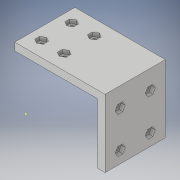
# Autodesk Inventor part: slotmountingPlate_dualcorner_m3
Saved by Autodesk Inventor 2018 (Build 220112000, 112)
## iProperties
Created: 2020-03-14
Part Number: slotmountingPlate_dualcorner_m3
Material: Generic
Document SubType Name: Modeling
Designer: natha
Density: 1 g/cm^3
Appearance: Default
Author: natha
Autodesk Inventor part; units mm, degrees
ref_plane "YZ Plane" through (0, 0, 0) normal (1, 0, 0) x (0, 1, 0)
ref_plane "XZ Plane" through (0, 0, 0) normal (0, 1, 0) x (-1, 0, 0)
ref_plane "XY Plane" through (0, 0, 0) normal (0, 0, 1) x (1, 0, 0)
sketch "Sketch1" plane through (0, 0, 0) normal (0, 1, 0) x (-1, 0, 0)
  line L0 (0, -5.4) -> (1.5, -5.4)
  line L1 (1.5, -5.4) -> (1.5, -8.1)
  line L2 (1.5, -8.1) -> (3.2, -8.1)
  line L3 (0, 0) -> (1.5, 0)
  line L4 (1.5, 0) -> (1.5, 2.7)
  line L5 (1.5, 2.7) -> (3.2, 2.7)
  line L6 (5, 0) -> (5, -5.4)
  line L7 (5, -5.4) -> (3.2, -8.1)
  line L8 (5, 0) -> (3.2, 2.7)
  line L9 (0, -20) -> (1.5, -20)
  line L10 (1.5, -20) -> (1.5, -17.3)
  line L11 (1.5, -17.3) -> (3.2, -17.3)
  line L12 (0, -25.4) -> (1.5, -25.4)
  line L13 (1.5, -25.4) -> (1.5, -28.1)
  line L14 (1.5, -28.1) -> (3.2, -28.1)
  line L15 (5, -20) -> (5, -25.4)
  line L16 (5, -25.4) -> (3.2, -28.1)
  line L17 (5, -20) -> (3.2, -17.3)
  line L18 (0, -5.4) -> (0, -20)
  line L19 (0, 0) -> (0, 7.3)
  line L20 (0, 7.3) -> (-5, 7.3)
  line L21 (0, -25.4) -> (0, -32.7)
  line L22 (0, -32.7) -> (-5, -32.7)
  line L23 (-5, -32.7) -> (-5, 7.3)
  dimension "d0" = 5.4
  dimension "d1" = 1.5
  dimension "d2" = 2.7
  dimension "d3" = 1.7
  dimension "d4" = 2.7
  dimension "d5" = 1.7
  dimension "d9" = 2.7
  dimension "d10" = 2.7
  dimension "d11" = 5.4
  dimension "d12" = 7.3
  dimension "d13" = 5
  dimension "d14" = 7.3
  dimension "d15" = 5
  dimension "d16" = 20
  constraints: 48 end point, 11 perpendicular, 4 vertical, 3 horizontal, 1 parallel
  measures "d0" distance of L3.start L0.start
  measures "d1" distance of L0.start L0.end
  measures "d2" distance of L0.end L1.end
  measures "d3" distance of L1.end L2.end
  measures "d4" distance of L3.end L4.end
  measures "d5" distance of L4.end L5.end
  measures "d9" distance of L9.end L10.end
  measures "d10" distance of L12.end L13.end
  measures "d11" distance between parallel lines of L12 L9
  measures "d12" distance of L3.start L19.end
  measures "d13" distance of L19.end L20.end
  measures "d14" distance of L12.start L21.end
  measures "d15" distance of L21.end L22.end
  measures "d16" distance between parallel lines of L3 L9
extrude "Extrusion1" add sketch "Sketch1" along normal blind 40
sketch "Sketch2" plane through (5, 0, 7.3) normal (1, 0, 0) x (0, 0, -1)
  line L0 (11.6599, 5) -> (8.3401, 5)
  line L1 (8.3401, 5) -> (6.6802, 7.875)
  line L2 (6.6802, 7.875) -> (8.3401, 10.75)
  line L3 (8.3401, 10.75) -> (11.6599, 10.75)
  line L4 (11.6599, 10.75) -> (13.3198, 7.875)
  line L5 (13.3198, 7.875) -> (11.6599, 5)
  line L6 (40, 0) -> (0, 0) projected
  line L7 (0, 0) -> (0, 40) projected
  line L8 (31.6599, 5) -> (28.3401, 5)
  line L9 (28.3401, 5) -> (26.6802, 7.875)
  line L10 (26.6802, 7.875) -> (28.3401, 10.75)
  line L11 (28.3401, 10.75) -> (31.6599, 10.75)
  line L12 (31.6599, 10.75) -> (33.3198, 7.875)
  line L13 (33.3198, 7.875) -> (31.6599, 5)
  line L14 (40, 0) -> (40, 40) projected
  line L15 (11.6599, 29.25) -> (8.3401, 29.25)
  line L16 (8.3401, 29.25) -> (6.6802, 32.125)
  line L17 (6.6802, 32.125) -> (8.3401, 35)
  line L18 (8.3401, 35) -> (11.6599, 35)
  line L19 (11.6599, 35) -> (13.3198, 32.125)
  line L20 (13.3198, 32.125) -> (11.6599, 29.25)
  line L21 (31.6599, 29.25) -> (28.3401, 29.25)
  line L22 (28.3401, 29.25) -> (26.6802, 32.125)
  line L23 (26.6802, 32.125) -> (28.3401, 35)
  line L24 (28.3401, 35) -> (31.6599, 35)
  line L25 (31.6599, 35) -> (33.3198, 32.125)
  line L26 (33.3198, 32.125) -> (31.6599, 29.25)
  line L27 (0, 40) -> (40, 40) projected
  point P0 (7.3, 0)
  point P1 (10, 7.875)
  point P2 (30, 7.875)
  point P3 (10, 32.125)
  point P4 (30, 32.125)
  dimension "d17" = 5.75
  dimension "d18" = 5
  dimension "d19" = 10
  dimension "d20" = 5.75
  dimension "d21" = 5
  dimension "d22" = 10
  dimension "d23" = 5.75
  dimension "d24" = 5.75
  dimension "d25" = 5
  dimension "d26" = 5
  dimension "d27" = 10
  dimension "d28" = 10
  constraints: 48 end point, 4 parallel, 52 other
  measures "d17" distance between parallel lines of L3 L0
  measures "d18" distance between parallel lines of L6 L0
  measures "d19" distance from line of L7 point (10, 7.875)
  measures "d20" distance between parallel lines of L11 L8
  measures "d21" distance between parallel lines of L6 L8
  measures "d22" distance from line of L14 point (30, 7.875)
  measures "d23" distance between parallel lines of L15 L18
  measures "d24" distance between parallel lines of L21 L24
  measures "d25" distance between parallel lines of L18 L27
  measures "d26" distance between parallel lines of L27 L24
  measures "d27" distance from line of L7 point (10, 32.125)
  measures "d28" distance from line of L14 point (30, 32.125)
extrude "Extrusion2" cut sketch "Sketch2" against normal blind 2.5 contours L0 L1 L2 L3 L4 L5 | L8 L9 L10 L11 L12 L13 | L15 L16 L17 L18 L19 L20 | L21 L22 L23 L24 L25 L26
sketch "Sketch3" plane through (2.5, 0, 7.3) normal (1, 0, 0) x (0, 0, -1)
  circle A0 centre (30, 7.75) radius 1.375
  circle A1 centre (10, 7.75) radius 1.375
  circle A2 centre (10, 32.25) radius 1.375
  circle A3 centre (30, 32.25) radius 1.375
  point P0 (7.3, 0)
  dimension "d31" = 2.75
  dimension "d32" = 2.75
  dimension "d33" = 2.75
  constraints: 4 centre point
  measures "d31" diameter of A0
  measures "d32" diameter of A1
  measures "d33" diameter of A2
extrude "Extrusion3" cut sketch "Sketch3" against normal blind 20
sketch "Sketch4" plane through (0, 40, 0) normal (0, 1, 0) x (1, 0, 0)
  line L0 (5, -7.3) -> (5, 32.7) projected
  line L1 (5, -7.3) -> (-55, -7.3)
  line L2 (-55, -7.3) -> (-55, 32.7)
  line L3 (-55, 32.7) -> (5, 32.7)
  line L4 (5, 32.7) -> (5, -7.3)
  point P0 (0, 0)
  dimension "d36" = 60
  constraints: 8 end point, 2 parallel, 1 horizontal, 1 perpendicular
  measures "d36" distance of L2.end L3.end
extrude "Extrusion4" add sketch "Sketch4" along normal blind 5
sketch "Sketch5" plane through (0, 40, 0) normal (0, -1, 0) x (1, 0, 0)
  line L0 (-55, -32.7) -> (-55, 7.3) projected
  line L1 (-20.2, 0) -> (-55, 0)
  line L2 (-55, 0) -> (-55, -5.4)
  line L3 (-55, -5.4) -> (-20.2, -5.4)
  line L4 (-20.2, -5.4) -> (-20.2, 0)
  line L5 (0, -5.4) -> (0, -20) projected
  line L6 (-20.2, -20) -> (-55, -20)
  line L7 (-55, -20) -> (-55, -25.4)
  line L8 (-55, -25.4) -> (-20.2, -25.4)
  line L9 (-20.2, -25.4) -> (-20.2, -20)
  point P0 (0, 0)
  dimension "d39" = 5.4
  dimension "d40" = 20.2
  dimension "d41" = 5.4
  constraints: 16 end point, 4 parallel, 2 horizontal, 2 perpendicular, 2 point on line
  measures "d39" distance of L2.end L1.end
  measures "d40" distance between parallel lines of L5 L4
  measures "d41" distance of L7.end L6.end
extrude "Extrusion5" add sketch "Sketch5" along normal blind 1.5
sketch "Sketch6" plane through (-55, 40, 7.3) normal (-1, 0, 0) x (0, 0, 1)
  point P0 (-7.3, -40)
sketch "Sketch7" plane through (-55, 40, 7.3) normal (-1, 0, 0) x (0, 0, 1)
  point P0 (-7.3, -40)
sketch "Sketch8" plane through (0, 38.5, 0) normal (0, -1, 0) x (1, 0, 0)
  line L0 (-55, -32.7) -> (-55, 7.3) projected
  line L1 (-20.2, 2.7) -> (-55, 2.7)
  line L2 (-55, 2.7) -> (-55, -8.1)
  line L3 (-55, -8.1) -> (-20.2, -8.1)
  line L4 (-20.2, -8.1) -> (-20.2, 2.7)
  line L5 (-20.2, -17.3) -> (-55, -17.3)
  line L6 (-55, -17.3) -> (-55, -28.1)
  line L7 (-55, -28.1) -> (-20.2, -28.1)
  line L8 (-20.2, -28.1) -> (-20.2, -17.3)
  line L9 (-20.2, -20) -> (-55, -20) projected
  point P0 (0, 0)
  dimension "d44" = 10.8
  dimension "d45" = 10.8
  dimension "d46" = 2.7
  constraints: 16 end point, 4 parallel, 3 point on line, 2 horizontal, 2 perpendicular
  measures "d44" distance of L2.end L1.end
  measures "d45" distance of L6.end L5.end
  measures "d46" distance between parallel lines of L9 L5
extrude "Extrusion6" add sketch "Sketch8" along normal blind 1.7 contours L0 L1 L4 L3 | L0 L9 L8 L7
sketch "Sketch9" plane through (-55, 40, 7.3) normal (-1, 0, 0) x (0, 0, 1)
  line L0 (-7.3, -4.809) -> (-12.7, -4.809)
  line L1 (-12.7, -40) -> (-12.7, 0) projected
  line L2 (-4.6, -3.2) -> (-15.4, -3.2) projected
  line L3 (-12.7, -4.809) -> (-15.4, -3.2)
  line L4 (-15.4, -3.2) -> (-4.6, -3.2)
  line L5 (-4.6, -3.2) -> (-7.3, -4.809)
  point P0 (-7.3, -40)
  dimension "d49" = 5.4
  constraints: 8 end point, 1 parallel, 1 point on line
  measures "d49" distance of L0.start L0.end
extrude "Extrusion7" add sketch "Sketch9" against normal blind 34.8
sketch "Sketch10" plane through (-55, 40, -20) normal (0, 0, 1) x (1, 0, 0)
  line L0 (34.8, -3.2) -> (0, -3.2) projected
  line L1 (0, 0) -> (0, -3.2) projected
  line L2 (34.8, -3.2) -> (0, -3.2)
  line L3 (0, -3.2) -> (0, -1.5)
  line L4 (0, -1.5) -> (34.8, -1.5)
  line L5 (34.8, -1.5) -> (34.8, -3.2)
  point P0 (55, -40)
  dimension "d52" = 1.7
  constraints: 8 end point, 2 parallel, 1 horizontal, 1 perpendicular, 1 point on line
  measures "d52" distance of L2.end L3.end
extrude "Extrusion8" add sketch "Sketch10" along normal blind 2.7
sketch "Sketch11" plane through (-55, 40, 7.3) normal (-1, 0, 0) x (0, 0, 1)
  line L0 (-24.6, -3.2) -> (-24.6, -1.5) projected
  line L1 (-35.4, -3.2) -> (-24.6, -3.2) projected
  line L2 (-24.6, -3.2) -> (-35.4, -3.2)
  line L3 (-27.3, -5) -> (-32.7, -5)
  line L4 (-32.7, -5) -> (-35.4, -3.2)
  line L5 (-24.6, -3.2) -> (-27.3, -5)
  line L6 (-27.3, 0) -> (-32.7, 0) projected
  point P0 (-7.3, -40)
  dimension "d55" = 5.4
  dimension "d56" = 5
  constraints: 8 end point, 2 horizontal
  measures "d55" distance of L3.start L3.end
  measures "d56" distance between parallel lines of L6 L3
extrude "Extrusion9" add sketch "Sketch11" against normal blind 34.8
sketch "Sketch12" plane through (0, 45, 0) normal (0, 1, 0) x (1, 0, 0)
  line L0 (-44.25, 4.3599) -> (-44.25, 1.0401)
  line L1 (-44.25, 1.0401) -> (-47.125, -0.6198)
  line L2 (-47.125, -0.6198) -> (-50, 1.0401)
  line L3 (-50, 1.0401) -> (-50, 4.3599)
  line L4 (-50, 4.3599) -> (-47.125, 6.0198)
  line L5 (-47.125, 6.0198) -> (-44.25, 4.3599)
  line L6 (-44.25, 24.3599) -> (-44.25, 21.0401)
  line L7 (-44.25, 21.0401) -> (-47.125, 19.3802)
  line L8 (-47.125, 19.3802) -> (-50, 21.0401)
  line L9 (-50, 21.0401) -> (-50, 24.3599)
  line L10 (-50, 24.3599) -> (-47.125, 26.0198)
  line L11 (-47.125, 26.0198) -> (-44.25, 24.3599)
  line L12 (-55, 25.4) -> (-20.2, 25.4) projected
  line L13 (-29.25, 4.3599) -> (-29.25, 1.0401)
  line L14 (-29.25, 1.0401) -> (-32.125, -0.6198)
  line L15 (-32.125, -0.6198) -> (-35, 1.0401)
  line L16 (-35, 1.0401) -> (-35, 4.3599)
  line L17 (-35, 4.3599) -> (-32.125, 6.0198)
  line L18 (-32.125, 6.0198) -> (-29.25, 4.3599)
  line L19 (-55, 32.7) -> (-55, -7.3) projected
  line L20 (5, 32.7) -> (-55, 32.7) projected
  line L21 (-55, -7.3) -> (5, -7.3) projected
  line L22 (-29.25, 24.3599) -> (-29.25, 21.0401)
  line L23 (-29.25, 21.0401) -> (-32.125, 19.3802)
  line L24 (-32.125, 19.3802) -> (-35, 21.0401)
  line L25 (-35, 21.0401) -> (-35, 24.3599)
  line L26 (-35, 24.3599) -> (-32.125, 26.0198)
  line L27 (-32.125, 26.0198) -> (-29.25, 24.3599)
  point P0 (0, 0)
  point P1 (-47.125, 2.7)
  point P2 (-47.125, 22.7)
  point P3 (-32.125, 2.7)
  point P4 (-32.125, 22.7)
  dimension "d59" = 5.75
  dimension "d60" = 5.75
  dimension "d61" = 5.75
  dimension "d62" = 5
  dimension "d63" = 5
  dimension "d64" = 20
  dimension "d67" = 10
  dimension "d69" = 10
  dimension "d70" = 10
  constraints: 48 end point, 3 parallel, 52 other
  measures "d59" distance between parallel lines of L3 L0
  measures "d60" distance between parallel lines of L9 L6
  measures "d61" distance between parallel lines of L16 L13
  measures "d62" distance between parallel lines of L19 L3
  measures "d63" distance between parallel lines of L19 L9
  measures "d64" distance between parallel lines of L19 L16
  measures "d67" distance from line of L20 point (-47.125, 22.7)
  measures "d69" distance from line of L21 point (-47.125, 2.7)
  measures "d70" distance from line of L21 point (-32.125, 2.7)
extrude "Extrusion10" cut sketch "Sketch12" against normal blind 2.5
sketch "Sketch13" plane through (0, 42.5, 0) normal (0, 1, 0) x (1, 0, 0)
  circle A0 centre (-47.125, 2.7) radius 1.375
  circle A1 centre (-32.125, 2.7) radius 1.375
  circle A2 centre (-47.125, 22.7) radius 1.375
  circle A3 centre (-32.125, 22.7) radius 1.375
  line L0 (-44.25, 4.3599) -> (-44.25, 1.0401) projected
  line L1 (-29.25, 4.3599) -> (-29.25, 1.0401) projected
  line L2 (-29.25, 24.3599) -> (-29.25, 21.0401) projected
  line L3 (-35, 24.3599) -> (-32.125, 26.0198) projected
  line L4 (-35, 4.3599) -> (-32.125, 6.0198) projected
  line L5 (-50, 4.3599) -> (-47.125, 6.0198) projected
  line L6 (-44.25, 24.3599) -> (-44.25, 21.0401) projected
  line L7 (-50, 24.3599) -> (-47.125, 26.0198) projected
  point P0 (0, 0)
  dimension "d73" = 2.75
  dimension "d74" = 2.75
  dimension "d75" = 2.75
  dimension "d76" = 2.75
  dimension "d77" = 2.875
  dimension "d78" = 2.875
  dimension "d79" = 2.875
  dimension "d80" = 2.875
  dimension "d81" = 2.875
  dimension "d82" = 2.875
  dimension "d83" = 2.875
  dimension "d84" = 2.875
  constraints: 4 centre point
  measures "d73" diameter of A0
  measures "d74" diameter of A1
  measures "d75" diameter of A2
  measures "d76" diameter of A3
  measures "d77" distance from line of A0.centre L0
  measures "d78" distance from line of A1.centre L1
  measures "d79" distance from line of L2 A3.centre
  measures "d80" distance from line of L3 A3.centre
  measures "d81" distance from line of L4 A1.centre
  measures "d82" distance from line of L5 A0.centre
  measures "d83" distance from line of A2.centre L6
  measures "d84" distance from line of L7 A2.centre
extrude "Extrusion11" cut sketch "Sketch13" against normal blind 20
body "Solid1"
